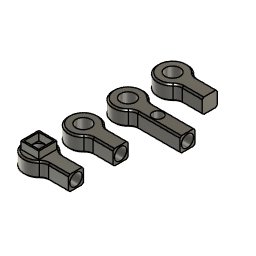
LinkHead (Autodesk Fusion 360 design; units mm, degrees)
part number: Configuration 1
Autodesk Fusion 360 part; units mm, degrees
note: some values were not read from the file. Set by a fixed rule: which sketch regions a step uses.
sketch "Sketch1" plane through (0, 0, 0) normal (0, 0, 1) x (1, 0, 0)
  circle A0 centre (0, 0) radius 10
  dimension "d7" = 20
  constraint coincident A0.centre origin
  measures "d7" diameter of A0
extrude "Extrude4" add sketch "Sketch1" along normal blind 10.1 makes body 1
sketch "Sketch6" plane through (0, 0, 0) normal (1, 0, 0) x (0, 1, 0)
  line L0 (10, 0) -> (-10, 0)
  line L1 (-5.05, 0) -> (5.05, 0)
  line L2 (5.05, 0) -> (5.05, 10.1)
  line L3 (5.05, 10.1) -> (-5.05, 10.1)
  line L4 (-5.05, 10.1) -> (-5.05, 0)
  dimension "d46" = 10.1
  dimension "d47" = 10.1
  constraint horizontal L1
  constraint vertical L2
  constraint horizontal L3
  constraint vertical L4
  constraint coincident L0 L1.start
  constraint midpoint origin L1
  measures "d46" distance of L1.start L1.end
  measures "d47" distance of L1.start L3.end
extrude "Extrude5" add sketch "Sketch6" along normal blind 25 bodies 1
sketch "Sketch7" plane through (25, 0, 0) normal (1, 0, 0) x (0, 1, 0)
  circle A0 centre (0, 5.1) radius 4.05
  line L0 (-5.05, 0) -> (5.05, 0)
  line L1 (-5.05, 10.1) -> (-5.05, 0)
  line L2 (5.05, 0) -> (5.05, 10.1)
  line L3 (5.05, 10.1) -> (-5.05, 10.1)
  dimension "d38" = 8.1
  measures "d38" diameter of A0
fillet "Fillet3" radius 6 2 edges at (8.6312, -5.05, 5.05) (8.6312, 5.05, 5.05) on bodies 1
chamfer "Chamfer3" distance 1 angle 45 10 edges at (-10, 0, 10.1) (9.2116, -5.5335, 10.1) (18.2857, -5.05, 10.1) (18.2857, 5.05, 10.1) (9.2116, 5.5335, 10.1) (-10, 0, 0) (9.2116, -5.5335, 0) (18.2857, -5.05, 0) (18.2857, 5.05, 0) (9.2116, 5.5335, 0) on bodies 1
sketch "Sketch9" plane through (0, 0, 10.1) normal (0, 0, 1) x (-1, 0, 0)
  line L0 (-25, -4.05) -> (-11.5714, -4.05)
  arc A0 (-6.5089, -6.2156) -> (-11.5714, -4.05) centre (-11.5714, -11.05) ccw
  arc A1 (-6.5089, -6.2156) -> (-6.5089, 6.2156) centre (0, 0) ccw
  arc A2 (-11.5714, 4.05) -> (-6.5089, 6.2156) centre (-11.5714, 11.05) ccw
  line L1 (-11.5714, 4.05) -> (-25, 4.05)
  line L2 (-25, 4.05) -> (-25, -4.05)
  circle A3 centre (0, 0) radius 5
  circle A4 centre (0, 0) radius 1.75
  dimension "d57" = 10
  dimension "d58" = 3.5
  constraint concentric A1 A3
  constraint coincident A1.centre A3.centre
  measures "d57" diameter of A3
  measures "d58" diameter of A4
extrude "Extrude10" cut sketch "Sketch9" against normal blind 10.2 contours A4 bodies 1
extrude "Extrude11" cut sketch "Sketch9" against normal blind 7.1 contours A3 bodies 1
copy_body "CopyPasteBodies1" bodies 1 makes body 2
move_body "Move1" bodies 2 to x (1, 0, 0) y (0, 1, 0) z (0, 0, 1) at (0, -30, 0)
sketch "Sketch10" plane through (0, 0, 0) normal (0, 0, -1) x (1, 0, 0)
  circle A0 centre (0, 30) radius 1.75
  line L0 (11.5714, 25.95) -> (25, 25.95)
  line L1 (25, 25.95) -> (25, 34.05)
  line L2 (25, 34.05) -> (11.5714, 34.05)
  arc A1 (6.5089, 36.2156) -> (11.5714, 34.05) centre (11.5714, 41.05) ccw
  arc A2 (6.5089, 36.2156) -> (6.5089, 23.7844) centre (0, 30) ccw
  arc A3 (11.5714, 25.95) -> (6.5089, 23.7844) centre (11.5714, 18.95) ccw
  circle A4 centre (20, 30) radius 1.5
  circle A5 centre (20, 30) radius 3.5
  dimension "d63" = 3
  dimension "d64" = 20
  dimension "d65" = 7
  constraint concentric A4 A5
  measures "d63" diameter of A4
  measures "d64" distance of A0.centre A4.centre
  measures "d65" diameter of A5
extrude "Extrude12" cut sketch "Sketch10" against normal blind 15 contours A4 bodies 2
extrude "Extrude13" cut sketch "Sketch10" along normal blind -29 and the other way blind 3 contours A5 bodies 2
extrude "Extrude14" add 1 faces at (25, -28.65, 6.7333) along direction (1, 0, 0) blind 15 on bodies 2 bodies 2
sketch "Sketch11" plane through (40, 0, 0) normal (1, 0, 0) x (0, 1, 0)
  line L0 (-25.95, 0) -> (-24.95, 1)
  line L1 (-24.95, 1) -> (-24.95, 9.1)
  line L2 (-24.95, 9.1) -> (-25.95, 10.1)
  line L3 (-25.95, 10.1) -> (-34.05, 10.1)
  line L4 (-34.05, 10.1) -> (-35.05, 9.1)
  line L5 (-35.05, 9.1) -> (-35.05, 1)
  line L6 (-35.05, 1) -> (-34.05, 0)
  line L7 (-34.05, 0) -> (-25.95, 0)
  circle A0 centre (-30, 5.05) radius 4.075
  line L8 (-24.95, 5.05) -> (-35.05, 5.05)
  point P0 (-30, 0)
  dimension "d74" = 8.15
  constraint vertical A0.centre P0
  constraint midpoint L1 L8.start
  constraint midpoint L5 L8.end
  constraint midpoint A0.centre L8
  measures "d74" diameter of A0
extrude "Extrude15" cut sketch "Sketch11" against normal blind 15 contours A0 L8 | A0 L8 bodies 2
copy_body "CopyPasteBodies2" bodies 1 makes body 3
move_body "Move2" bodies 3 to x (1, 0, 0) y (0, 1, 0) z (0, 0, 1) at (0, -60, 0)
sketch "Sketch12" plane through (25, 0, 0) normal (1, 0, 0) x (0, 1, 0)
  line L0 (-55.95, 0) -> (-54.95, 1)
  line L1 (-54.95, 1) -> (-54.95, 9.1)
  line L2 (-54.95, 9.1) -> (-55.95, 10.1)
  line L3 (-55.95, 10.1) -> (-64.05, 10.1)
  line L4 (-64.05, 10.1) -> (-65.05, 9.1)
  line L5 (-65.05, 9.1) -> (-65.05, 1)
  line L6 (-65.05, 1) -> (-64.05, 0)
  line L7 (-64.05, 0) -> (-55.95, 0)
  line L8 (-65.05, 5.05) -> (-54.95, 5.05)
  circle A0 centre (-60, 5.05) radius 4.125
  dimension "d77" = 8.25
  constraint midpoint L5 L8.start
  constraint midpoint L1 L8.end
  constraint midpoint L8 A0.centre
  measures "d77" diameter of A0
extrude "Extrude16" cut sketch "Sketch12" against normal blind 15 contours L8 A0 | L8 A0 bodies 3
copy_body "CopyPasteBodies3" bodies 3 makes body 4
move_body "Move3" bodies 4 to x (1, 0, 0) y (0, 1, 0) z (0, 0, 1) at (0, -30, 0)
sketch "Sketch13" plane through (0, 0, 10.1) normal (0, 0, 1) x (-1, 0, 0)
  circle A0 centre (0, 90) radius 5
  line L0 (-25, 85.95) -> (-11.5714, 85.95)
  arc A1 (-6.5089, 83.7844) -> (-11.5714, 85.95) centre (-11.5714, 78.95) ccw
  arc A2 (-6.5089, 83.7844) -> (-6.5089, 96.2156) centre (0, 90) ccw
  arc A3 (-11.5714, 94.05) -> (-6.5089, 96.2156) centre (-11.5714, 101.05) ccw
  line L1 (-11.5714, 94.05) -> (-25, 94.05)
  line L2 (-25, 94.05) -> (-25, 85.95)
  line L3 (-6, 96) -> (6, 96)
  line L4 (6, 96) -> (6, 84)
  line L5 (6, 84) -> (-6, 84)
  line L6 (-6, 84) -> (-6, 96)
  line L7 (-6, 96) -> (6, 84) construction
  line L8 (6, 96) -> (-6, 84) construction
  line L9 (-5, 95) -> (5, 95)
  line L10 (5, 95) -> (5, 85)
  line L11 (5, 85) -> (-5, 85)
  line L12 (-5, 85) -> (-5, 95)
  point P0 (0, 90)
  dimension "d80" = 12
  dimension "d81" = 12
  dimension "d82" = 1
  constraint horizontal L3
  constraint perpendicular L3 L4
  constraint parallel L3 L5
  constraint parallel L4 L6
  constraint coincident L7 P0
  constraint coincident L8 P0
  constraint coincident P0 A0.centre
  measures "d80" distance of L4.end L5.end
  measures "d81" distance of L3.end L4.end
extrude "Extrude17" add sketch "Sketch13" along normal blind 5 contours L3 L4 L5 L6 bodies 4
copy_body "CopyPasteBodies4" bodies 2 makes body 5
move_body "Move4" bodies 5 to x (1, 0, 0) y (0, 1, 0) z (0, 0, 1) at (328, 0, 0)
move_body "Move5" bodies 5 to x (-1, 0, 0) y (0, -1, 0) z (0, 0, 1) at (656, -60, 0)
hidden bodies 5
equation "HeadDia = 20 mm"
equation "HoleDia = 3.5 mm"
equation "ConLength = 15 mm"
equation "WallTh = 1 mm"
equation "ProfileDia = 8.1 mm"
equation "d7 = HeadDia"
equation "ConTh = ProfileDia + 2 * WallTh"
equation "d17 = HeadDia"
equation "d30 = ConTh"
equation "d34 = ConLength + HeadDia / 2"
equation "d38 = ProfileDia"
equation "Chamfer = 1 mm"
equation "d46 = ConTh"
equation "d47 = ConTh"
equation "d50 = Chamfer"
equation "d61 = -ConTh + 3 mm"
equation "d72 = ConLength"
equation "d75 = -ConLength"
equation "d78 = -ConLength"
named bodies: "Base", "ServoLinkHead", "Base (1)", "BaseHead", "BaseHead (1)", "ServoLinkHead (1)"
